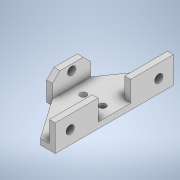
# Autodesk Inventor part: Part3
Saved by Autodesk Inventor 2022 (Build 260153000, 153)
## iProperties
Created: 2022-12-27
Part Number: Part3
Material: Generic
Document SubType Name: Modeling
Designer: Gaming
Density: 1 g/cm^3
Appearance: Default
Author: Gaming
Autodesk Inventor part; units mm, degrees
ref_plane "YZ Plane" through (0, 0, 0) normal (1, 0, 0) x (0, 1, 0)
ref_plane "XZ Plane" through (0, 0, 0) normal (0, 1, 0) x (-1, 0, 0)
ref_plane "XY Plane" through (0, 0, 0) normal (0, 0, 1) x (1, 0, 0)
sketch "Sketch1" plane through (0, 0, 0) normal (0, 0, 1) x (1, 0, 0)
  line L0 (0, 0) -> (-29, 0)
  line L1 (-29, 0) -> (-29, 4)
  line L2 (-29, 4) -> (-4, 4)
  line L3 (-4, 4) -> (-4, 18)
  line L4 (-4, 18) -> (0, 18)
  line L5 (0, 18) -> (0, 0)
  dimension "d0" = 4
  dimension "d1" = 4
  dimension "d2" = 29
  dimension "d3" = 18
  constraints: 12 end point, 5 perpendicular, 1 horizontal
  measures "d0" distance of L3.end L4.end
  measures "d1" distance between parallel lines of L0 L2
  measures "d2" distance between parallel lines of L1 L5
  measures "d3" distance between parallel lines of L0 L4
extrude "Extrusion1" add sketch "Sketch1" along normal blind 80
sketch "Sketch2" plane through (0, 0, 0) normal (1, 0, 0) x (0, 0, -1)
  line L0 (0, 4) -> (-80, 4) projected
  line L1 (-51, 18) -> (-29, 18)
  line L2 (-29, 18) -> (-29, 4)
  line L3 (-29, 4) -> (-51, 4)
  line L4 (-51, 4) -> (-51, 18)
  line L5 (0, 18) -> (-80, 18) projected
  point P0 (0, 0)
  point P1 (-40, 18)
  point P2 (-40, 4)
  point P3 (-51, 4)
  dimension "d6" = 22
  constraints: 8 end point, 2 midpoint, 2 parallel, 1 collinear, 1 horizontal, 1 perpendicular, 1 point on line, 1 vertical alignment
  measures "d6" distance between parallel lines of L4 L2
extrude "Extrusion2" cut sketch "Sketch2" against normal through all
sketch "Sketch3" plane through (0, 0, 0) normal (1, 0, 0) x (0, 0, -1)
  line L0 (0, 0) -> (-80, 0) projected
  line L1 (-80, 0) -> (-80, 18) projected
  line L2 (0, 0) -> (0, 18) projected
  point P0 (-70, 9)
  point P1 (-10, 9)
  dimension "d9" = 9
  dimension "d10" = 10
  dimension "d11" = 10
  constraints: 1 horizontal alignment
  measures "d9" distance from line of point (-70, 9) L0
  measures "d10" distance from line of point (-70, 9) L1
  measures "d11" distance from line of point (-10, 9) L2
hole "Hole1" at (0, 9, 70) at (0, 9, 10) direction (-1, 0, 0) diameter 5.5 end through all
sketch "Sketch4" plane through (-29, 0, 0) normal (0, -1, 0) x (1, 0, 0)
  line L0 (29, 0) -> (29, 80) projected
  line L1 (0, 0) -> (29, 0) projected
  point P0 (20, 60)
  point P1 (20, 20)
  dimension "d19" = 9
  dimension "d20" = 20
  dimension "d21" = 20
  constraints: 1 vertical alignment
  measures "d19" distance from line of point (20, 60) L0
  measures "d20" vertical distance of point (20, 60) L0.end
  measures "d21" distance from line of point (20, 20) L1
hole "Hole2" at (-9, 0, 60) at (-9, 0, 20) direction (0, 1, 0) diameter 5.5 end through all
sketch "Sketch5" plane through (-29, 4, 0) normal (0, 1, 0) x (1, 0, 0)
  line L0 (0, 0) -> (0, -80) projected
  line L1 (0, -52.8652) -> (19, -80)
  line L2 (25, -80) -> (0, -80) projected
  line L3 (25, 0) -> (0, 0) projected
  line L4 (19, 0) -> (0, -27.1348)
  line L5 (25, -29) -> (29, -29) projected
  line L6 (29, -51) -> (25, -51) projected
  line L7 (29, -51) -> (29, -80) projected
  line L8 (29, 0) -> (29, -29) projected
  dimension "d29" = 10
  dimension "d30" = 10
  dimension "d31" = 55
  dimension "d32" = 55
  constraints: 4 end point, 4 point on line
  measures "d29" distance from line of L1.end L7
  measures "d30" distance from line of L4.start L8
  measures "d31" angle of L4 L3
  measures "d32" angle of L2 L1
extrude "Extrusion3" cut sketch "Sketch5" against normal through all
sketch "Sketch6" plane through (-4, 4, 51) normal (0, 1, 0) x (1, 0, 0)
  line L0 (4, 22) -> (4, 0) projected
  line L1 (-25, 23.8652) -> (-25, -1.8652) projected
  point P0 (4, 51)
  point P1 (-4, 11)
  point P2 (-17, 11)
  point P3 (-25, 11)
  dimension "d35" = 8
  dimension "d36" = 8
  constraints: 2 horizontal alignment, 1 midpoint
  measures "d35" distance from line of point (-4, 11) L0
  measures "d36" distance from line of point (-17, 11) L1
hole "Hole3" at (-8, 4, 40) at (-21, 4, 40) direction (0, -1, 0) diameter 4.5 end through all
sketch "Sketch7" plane through (-29, 0, 27.1348) normal (-1, 0, 0) x (0, 0, 1)
  line L0 (0, 4) -> (0, 0) projected
  line L1 (0, 0) -> (25.7304, 0) projected
  line L2 (25.7304, 0) -> (25.7304, 4) projected
  line L3 (0, 4) -> (25.7304, 4) projected
  line L4 (0, 0) -> (25.7304, 0)
  line L5 (25.7304, 0) -> (25.7304, 18)
  line L6 (25.7304, 18) -> (0, 18)
  line L7 (0, 18) -> (0, 0)
  line L8 (25.7304, 0) -> (25.7304, 4) projected
  line L9 (-27.1348, 18) -> (1.8652, 18) projected
  point P0 (-27.1348, 0)
  constraints: 8 end point, 2 collinear, 2 parallel, 1 horizontal, 1 perpendicular
extrude "Extrusion4" add sketch "Sketch7" along normal blind 4
sketch "Sketch8" plane through (-33, 0, 27.1348) normal (-1, 0, 0) x (0, 0, 1)
  line L0 (25.7304, 18) -> (0, 18) projected
  line L1 (-27.1348, 4) -> (0, 4) projected
  point P0 (-27.1348, 0)
  point P1 (12.8652, 14)
  point P2 (12.8652, 18)
  dimension "d46" = 10
  constraints: 1 midpoint, 1 vertical alignment
  measures "d46" distance from line of point (12.865, 14) L1
hole "Hole4" at (-33, 14, 40) direction (1, 0, 0) diameter 5.5 end through all
chamfer "Chamfer1" distance 5 angle 45 2 edges at (-31, 18, 27.1348) (-31, 18, 52.8652)
equation "\"d11\" = d10"
equation "\"d21\" = d20"
equation "\"d30\" = d29"
equation "\"d32\" = d31"
equation "\"d36\" = d35"
body "Solid1"
